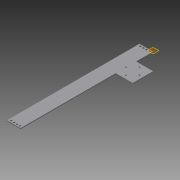
# Autodesk Inventor part: Cim Mount
Saved by Autodesk Inventor 2013 (Build 170138000, 138)
## iProperties
Created: 2013-01-24
Part Number: Cim Mount
Material: Aluminum 6061
Document SubType Name: Modeling
Designer: actoennies
Density: 2.71 g/cm^3
Mass: 254.955 g
Surface Area: 638.763 cm^2
Volume: 94.0792 cm^3
Author: actoennies
Autodesk Inventor part; units mm, degrees
ref_plane "YZ Plane" through (0, 0, 0) normal (1, 0, 0) x (0, 1, 0)
ref_plane "XZ Plane" through (0, 0, 0) normal (0, 1, 0) x (-1, 0, 0)
ref_plane "XY Plane" through (0, 0, 0) normal (0, 0, 1) x (1, 0, 0)
sketch "Sketch1" plane through (0, 0, 0) normal (0, 1, 0) x (-1, 0, 0)
  line L0 (0, 0) -> (0, 63.5)
  line L1 (0, 63.5) -> (-63.5, 63.5)
  line L2 (-63.5, 63.5) -> (-63.5, 139.7)
  line L3 (-63.5, 139.7) -> (0, 139.7)
  line L4 (0, 139.7) -> (0, 495.3)
  line L5 (0, 495.3) -> (50.8, 495.3)
  line L6 (50.8, 495.3) -> (50.8, 0)
  line L7 (50.8, 0) -> (0, 0)
  circle A0 centre (-25.4, 101.6) radius 25.4 construction
  circle A1 centre (-25.4, 127) radius 2.5527
  circle A2 centre (-50.8, 101.6) radius 2.5527
  circle A3 centre (-25.4, 76.2) radius 2.5527
  circle A4 centre (0, 101.6) radius 2.5527
  dimension "d6" = 50.8
  dimension "d1" = 63.5
  dimension "d2" = 63.5
  dimension "d3" = 76.2
  dimension "d4" = 355.6
  dimension "d5" = 50.8
  dimension "d30" = 101.6
  dimension "d31" = 38.1
  dimension "d32" = 5.1054
  dimension "d35" = 360
  constraints: 16 end point, 4 centre point, 4 perpendicular, 3 parallel, 1 vertical, 1 vertical alignment, 11 other
  measures "d1" distance of L0.start L0.end
  measures "d2" distance of L0.end L1.end
  measures "d3" distance of L1.end L2.end
  measures "d4" distance of L3.end L4.end
  measures "d5" distance of L4.end L5.end
  measures "d30" distance from line of L7 point (-25.4, 101.6)
  measures "d31" distance from line of L2 point (-25.4, 101.6)
  measures "d32" diameter of A1
ref_plane "Work Plane2" through (0, 6.35, 0) normal (0, 1, 0) x (1, 0, 0)
ref_plane "Work Plane1" through (0, 6.35, 0) normal (0, 1, 0) x (1, 0, 0)
extrude "Extrusion4" add sketch "Sketch1" along normal blind 3.175
sketch "Sketch5" plane through (0, 3.175, 0) normal (0, 1, 0) x (1, 0, 0)
  circle A0 centre (-7.8014, -488.95) radius 3.3782 projected
  circle A1 centre (-18.8686, -488.95) radius 3.3782 projected
  circle A2 centre (-29.9357, -488.95) radius 3.3782 projected
  circle A3 centre (-41.0029, -488.95) radius 3.3782 projected
  circle A4 centre (-7.8014, -6.35) radius 3.3782 projected
  circle A5 centre (-41.0029, -6.35) radius 3.3782 projected
  circle A6 centre (-29.9357, -6.35) radius 3.3782 projected
  circle A7 centre (-18.8686, -6.35) radius 3.3782 projected
extrude "Extrusion6" cut sketch "Sketch5" against normal blind 25.4
body "Solid1"
